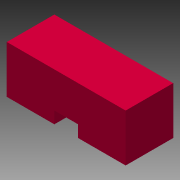
# Autodesk Inventor part: block
Saved by Autodesk Inventor 2015 (Build 190159000, 159)
## iProperties
Created: 2017-04-05
Part Number: block
Material: Generic
Document SubType Name: Modeling
Designer: Mohalla
Density: 1 g/cm^3
Appearance: Default
Mass: 19 g
Surface Area: 49 cm^2
Volume: 19 cm^3
Author: Mohalla
Autodesk Inventor part; units mm, degrees
ref_plane "YZ Plane" through (0, 0, 0) normal (1, 0, 0) x (0, 1, 0)
ref_plane "XZ Plane" through (0, 0, 0) normal (0, 1, 0) x (-1, 0, 0)
ref_plane "XY Plane" through (0, 0, 0) normal (0, 0, 1) x (1, 0, 0)
sketch "Sketch1" plane through (0, 0, 0) normal (0, 0, 1) x (1, 0, 0)
  line L0 (-25, 20) -> (25, 20)
  line L1 (25, 20) -> (25, 0)
  line L2 (-25, 0) -> (-25, 20)
  line L3 (-25, 0) -> (-5, 0)
  line L4 (-5, 0) -> (-5, 5)
  line L5 (-5, 5) -> (5, 5)
  line L6 (5, 5) -> (4.4322, 5)
  line L7 (5, 5) -> (5, 0)
  line L8 (5, 0) -> (25, 0)
  point P0 (0, 0)
  dimension "d0" = 50
  dimension "d1" = 20
  dimension "d3" = 25
  dimension "d4" = 20
  dimension "d5" = 5
  dimension "d6" = 10
  dimension "d7" = 5
  dimension "d8" = 20
  constraints: 18 end point, 4 perpendicular, 2 horizontal, 2 point on line, 1 parallel
  measures "d0" distance of L0.start L0.end
  measures "d1" distance of L2.start L0.start
  measures "d3" distance from line of point (0, 0) L2
  measures "d4" distance of L2.start L3.end
  measures "d5" distance of L3.end L4.end
  measures "d6" distance of L4.end L5.end
  measures "d7" distance of L5.end L7.end
  measures "d8" distance from line of point (0, 0) L0
extrude "Extrusion1" add sketch "Sketch1" along normal mid plane 20
body "Solid1"
